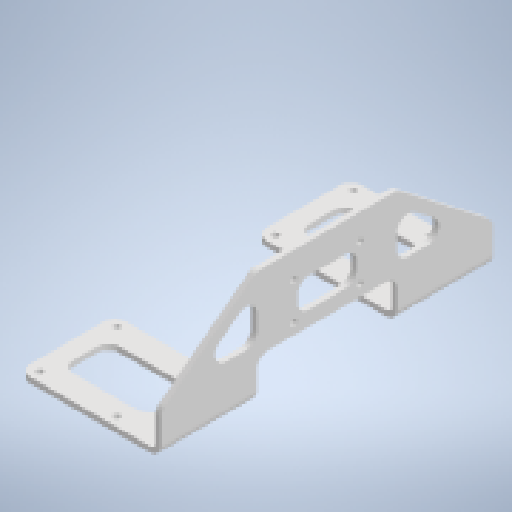
# Autodesk Inventor part: hipjoint_front
Saved by Autodesk Inventor 2024.1 (Build 281209000, 209)
## iProperties
Created: 2024-10-08
Part Number: hipjoint_front
Material: 一般
Document SubType Name: Sheet Metal
Designer: hibik
Density: 1 g/cm^3
Sheet Metal Rule: Default_mm
Appearance: 既定
Flat Pattern Width: 6.68929 cm
Flat Pattern Length: 9 cm
Flat Pattern Area: 60.2036 cm^2
Sheet Metal Width: 66.893 mm
Sheet Metal Length: 90.000 mm
Sheet Metal Area: 6020.363 mm^2
Author: hibik
Autodesk Inventor part; units mm, degrees
note: some values were not read from the file. Chosen so that the rebuilt part matches the saved one: flange form of "プレート3".
ref_plane "YZ Plane" through (0, 0, 0) normal (1, 0, 0) x (0, 1, 0)
ref_plane "XZ Plane" through (0, 0, 0) normal (0, 1, 0) x (-1, 0, 0)
ref_plane "XY Plane" through (0, 0, 0) normal (0, 0, 1) x (1, 0, 0)
sketch "スケッチ2" plane through (0, 0, 0) normal (0, 1, 0) x (-1, 0, 0)
  line L0 (0, 0) -> (24, 0)
  line L1 (24, 0) -> (24, -26)
  line L2 (24, -26) -> (0, -26)
  line L3 (0, -26) -> (0, 0)
  circle A0 centre (0, -13) radius 6.25
  line L4 (0, 0) -> (-14.5, 0)
  line L5 (-14.5, 0) -> (-14.5, -26)
  line L6 (-14.5, -26) -> (0, -26)
  line L7 (0, -26) -> (0, 0)
  line L8 (0, -6.75) -> (19, -6.75)
  line L9 (19, -6.75) -> (19, -19.25)
  line L10 (19, -19.25) -> (0, -19.25)
  line L11 (0, -19.25) -> (0, -6.75)
  point P0 (0, -6.75)
  point P1 (0, -19.25)
  point P2 (0, -6.75)
  point P3 (0, -19.25)
  dimension "d1" = 12.5
  dimension "d0" = 26
  dimension "d2" = 24
  dimension "d14" = 14.5
  dimension "d32" = 5
  measures "d0" distance of L0.end L1.end
  measures "d2" distance of L0.start L0.end
  measures "d14" distance between parallel lines of L3 L5
  measures "d32" distance between parallel lines of L1 L9
extrude "プレート1" add sketch "スケッチ2" along normal blind 1.5 contours L0 L1 L2 L3 L10 L9 L8 | L3 A0 L6 L5 L4
sketch "スケッチ4" plane through (13, 0, -26) normal (1, 0, 0) x (0, 1, 0)
  line L0 (0, 26) -> (0, 0)
  line L1 (0, 0) -> (31, 0)
  line L2 (31, 0) -> (31, 26)
  line L3 (31, 26) -> (0, 26)
  constraints: 6 end point, 1 horizontal, 1 perpendicular, 1 vertical
edge flange "フランジ2" height 31 angle 90 thickness 1.5 bend radius 1.5 thickness toward (1, 0, 0) relief tear relief width 1.5 relief depth 0.75 edges at (14.5, 1.5, -13) wall of the first edge with corners at (13, 0, 0) (13, 0, -26) (13, 31, -26) (13, 31, 0)
bend "曲げ2"
corner "コーナー2"
sketch "スケッチ5" plane through (14.5, 31, 0) normal (1, 0, 0) x (0, 0, -1)
  line L0 (0, -28) -> (0, 0)
  line L1 (0, 0) -> (45, 0)
  line L2 (45, 0) -> (45, -20)
  line L3 (45, -20) -> (0, -20)
  line L4 (0, -20) -> (0, 0)
  point P0 (0, -31)
  point P1 (0, -20)
  dimension "d25" = 20
  dimension "d26" = 45
  measures "d25" distance of L1.end L2.end
  measures "d26" distance of L2.end L3.end
sheet face with bend "面2" sketch "スケッチ5" thickness 1.5 toward (-1, 0, 0) bend radius 1.5
bend "曲げ3"
mirror "ミラー1" about plane through (14.5, 11, -45) normal (0, 0, -1)
sketch "スケッチ6" plane through (0, 0, 0) normal (0, -1, 0) x (1, 0, 0)
  circle A0 centre (0, -2.5) radius 0.85 projected
  circle A1 centre (0, -23.5) radius 0.85 projected
  circle A2 centre (-21, -23.5) radius 0.85 projected
  circle A3 centre (-21, -2.5) radius 0.85 projected
  circle A4 centre (0, -66.5) radius 0.85 projected
  circle A5 centre (0, -87.5) radius 0.85 projected
  circle A6 centre (-21, -87.5) radius 0.85 projected
  circle A7 centre (-21, -66.5) radius 0.85 projected
  point P0 (0, 0)
extrude "切り取り1" cut sketch "スケッチ6" against normal blind 1.5
sketch "スケッチ7" plane through (14.5, 3, 0) normal (1, 0, 0) x (0, 0, -1)
  circle A0 centre (36, 21) radius 0.8 projected
  circle A1 centre (36, 11) radius 0.8 projected
  circle A2 centre (54, 11) radius 0.8 projected
  circle A3 centre (54, 21) radius 0.8 projected
  line L0 (53, 17) -> (53, 15) projected
  arc A4 (53, 17) -> (50, 20) centre (50, 17) ccw projected
  line L1 (40, 20) -> (50, 20) projected
  arc A5 (40, 20) -> (37, 17) centre (40, 17) ccw projected
  line L2 (37, 15) -> (37, 17) projected
  arc A6 (37, 15) -> (40, 12) centre (40, 15) ccw projected
  line L3 (50, 12) -> (40, 12) projected
  arc A7 (50, 12) -> (53, 15) centre (50, 15) ccw projected
  line L4 (0, 0) -> (0, 28) projected
  line L5 (0, 0) -> (26, 0) projected
  line L6 (26, 8) -> (26, 0) projected
  line L7 (26, 8) -> (64, 8) projected
  line L8 (64, 8) -> (64, 0) projected
  line L9 (90, 0) -> (64, 0) projected
  line L10 (90, 0) -> (90, 28) projected
  line L11 (90, 28) -> (0, 28) projected
  line L12 (0, 8) -> (26, 28)
  line L13 (64, 28) -> (90, 8)
  line L14 (26, 24.2151) -> (26, 11)
  line L15 (26, 11) -> (8.8204, 11)
  line L16 (8.8204, 11) -> (26, 24.2151)
  line L17 (64, 24.2151) -> (64, 11)
  line L18 (64, 11) -> (81.1796, 11)
  line L19 (81.1796, 11) -> (64, 24.2151)
  line L20 (8.8204, 8) -> (23, 8)
  line L21 (23, 8) -> (23, 3)
  line L22 (23, 3) -> (8.8204, 3)
  line L23 (8.8204, 3) -> (8.8204, 8)
  line L24 (67, 8) -> (81.1796, 8)
  line L25 (81.1796, 8) -> (81.1796, 3)
  line L26 (81.1796, 3) -> (67, 3)
  line L27 (67, 3) -> (67, 8)
  point P0 (0, -3)
  dimension "d37" = 3
  dimension "d38" = 3
  dimension "d39" = 3
  dimension "d40" = 3
  dimension "d41" = 3
  dimension "d42" = 3
  dimension "d43" = 3
  constraints: 32 end point, 9 point on line, 7 parallel, 5 collinear, 2 horizontal, 2 perpendicular, 1 horizontal alignment, 1 vertical
  measures "d37" distance between parallel lines of L15 L7
  measures "d38" distance between parallel lines of L12 L16
  measures "d39" distance between parallel lines of L13 L19
  measures "d40" distance between parallel lines of L6 L21
  measures "d41" distance between parallel lines of L8 L27
  measures "d42" distance between parallel lines of L5 L22
  measures "d43" distance between parallel lines of L26 L9
extrude "切り取り2" cut sketch "スケッチ7" against normal blind 1.5 contours A0 | A1 | A2 | A3 | L0 A7 L3 A6 L2 A5 L1 A4 | L4 L11 L12 | L11 L10 L13 | L14 L15 L16 | L19 L18 L17
fillet "フィレット1" radius 3 20 edges at (13.75, 27.2151, -26) (13.75, 14, -26) (13.75, 14, -8.8204) (13.75, 31, -26) (13.75, 11, 0) (13.75, 31, -64) (13.75, 11, -90) (13.75, 11, -64) (13.75, 11, -26) (13.75, 14, -64) (13.75, 27.2151, -64) (13.75, 14, -81.1796) (-19, 0.75, -6.75) (-19, 0.75, -19.25) (-19, 0.75, -70.75) (-19, 0.75, -83.25) (-24, 0.75, -90) (-24, 0.75, -64) (-24, 0.75, -26) (-24, 0.75, 0)
equation "\"d33\" = Thickness"
equation "\"d39\" = d38"
equation "\"d40\" = d37"
equation "\"d41\" = d40"
equation "\"d42\" = d37"
equation "\"d43\" = d37"
equation "\"d35\" = Thickness"
equation "\"d3\" = Thickness"
equation "\"d15\" = BendReliefWidth"
equation "\"d16\" = BendReliefDepth"
equation "\"d17\" = MinimumRemnant"
equation "\"d18\" = TransitionRadius"
equation "\"d21\" = BendRadius"
equation "\"d22\" = CornerReliefSize"
equation "\"d23\" = GapSize"
equation "\"d24\" = JacobiRadiusSize"
equation "\"d27\" = BendRadius"
equation "\"d28\" = BendReliefWidth"
equation "\"d30\" = MinimumRemnant"
equation "\"d29\" = BendReliefDepth"
equation "\"d31\" = TransitionRadius"
equation "\"BendRadius\" = Thickness"
equation "\"BendReliefWidth\" = Thickness"
equation "\"BendReliefDepth\" = 0.5 * Thickness"
equation "\"CornerReliefSize\" = 4 * Thickness"
equation "\"MinimumRemnant\" = 2 * Thickness"
equation "\"TransitionRadius\" = BendRadius"
equation "\"JacobiRadiusSize\" = BendRadius"
equation "\"GapSize\" = Thickness"
equation "\"Thickness\" = 1.5"
